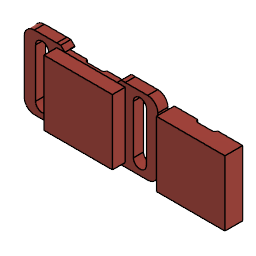
LeverSensor (Autodesk Fusion 360 design; units mm, degrees)
Autodesk Fusion 360 part; units mm, degrees
note: some values were not read from the file. Set by a fixed rule: which sketch regions a step uses.
sketch "Sketch1" plane through (0, 0, 0) normal (0, 0, 1) x (1, 0, 0)
  line L0 (0, 0) -> (12.8, 0)
  line L1 (12.8, 0) -> (12.8, 5.8)
  line L2 (12.8, 5.8) -> (0, 5.8)
  line L3 (0, 5.8) -> (0, 0)
  dimension "d1" = 12.8
  dimension "d2" = 5.8
  constraint horizontal L0
  constraint vertical L1
  constraint horizontal L2
  constraint vertical L3
  constraint coincident L0.start L3.end
  measures "d1" distance of L0.start L0.end
  measures "d2" distance of L0.start L2.end
extrude "Extrude1" add sketch "Sketch1" along normal blind 6 makes body 1
sketch "Sketch2" plane through (0, 0, 0) normal (0, -1, 0) x (1, 0, 0)
  line L0 (0, 0) -> (12.8, 0)
  line L1 (12.8, 0) -> (12.8, 6)
  line L2 (12.8, 6) -> (0, 6)
  line L3 (0, 6) -> (0, 0)
  line L4 (0, 4.8) -> (3.2, 4.8) construction
  circle A0 centre (3.2, 4.8) radius 1.2
  line L5 (6.4, 6) -> (6.4, 0) construction
  circle A1 centre (9.6, 4.8) radius 1.2
  line L6 (1.6, 4.8) -> (4, 4.8)
  line L7 (4, 4.8) -> (4, 6.5)
  line L8 (4, 6.5) -> (1.6, 6.5)
  line L9 (1.6, 6.5) -> (1.6, 4.8)
  line L10 (11.2, 6.5) -> (11.2, 4.8)
  line L11 (11.2, 4.8) -> (8.8, 4.8)
  line L12 (8.8, 4.8) -> (8.8, 6.5)
  line L13 (8.8, 6.5) -> (11.2, 6.5)
  dimension "d5" = 3.2
  dimension "d6" = 2.4
  dimension "d7" = 2.4
  dimension "d8" = 1.7
  constraint coincident L3 L4.start
  constraint perpendicular L3 L4
  constraint coincident L4.end A0.centre
  constraint midpoint L2 L5.start
  constraint midpoint L0 L5.end
  constraint symmetric A0 L5 A1
  constraint horizontal L6
  constraint vertical L7
  constraint horizontal L8
  constraint vertical L9
  constraint midpoint L4 L6.start
  constraint symmetric L5 L6.start L10.end
  constraint symmetric L5 L6.end L11.end
  constraint symmetric L5 L7.end L12.end
  constraint symmetric L5 L8.end L10.start
  measures "d5" distance of L4.start L4.end
  measures "d6" diameter of A0
  measures "d7" distance of L6.start L6.end
  measures "d8" distance of L6.start L8.end
extrude "Extrude2" cut sketch "Sketch2" against normal blind 12 contours A0 L6 L7 | A1 L11 L12 | A0 L6 L7 | A1 L11 L12 bodies 1
extrude "Extrude3" add sketch "Sketch2" against normal blind 5.8 contours L2 L7 L8 L9 | L2 L10 L12 L13 bodies 1
chamfer "Chamfer1" distance 0.5 angle 45 4 edges at (11.2, 2.9, 6.5) (4, 2.9, 6.5) (8.8, 2.9, 6.5) (1.6, 2.9, 6.5) on bodies 1
sketch "Sketch3" plane through (0, 0, 6) normal (0, 0, 1) x (-1, 0, 0)
  line L0 (-8.8, 0) -> (-8.8, -5.8)
  line L1 (-8.8, -5.8) -> (-4, -5.8)
  line L2 (-4, -5.8) -> (-4, 0)
  line L3 (-4, 0) -> (-8.8, 0)
  line L4 (-6.15, -2.65) -> (-6.65, -2.65)
  line L5 (-6.65, -2.65) -> (-6.65, -3.15)
  line L6 (-6.65, -3.15) -> (-6.15, -3.15)
  line L7 (-6.15, -3.15) -> (-6.15, -2.65)
  line L8 (-6.15, -2.65) -> (-6.65, -3.15) construction
  line L9 (-6.65, -2.65) -> (-6.15, -3.15) construction
  line L10 (-11.7603, -2.65) -> (-12.2603, -2.65)
  line L11 (-12.2603, -2.65) -> (-12.2603, -3.15)
  line L12 (-12.2603, -3.15) -> (-11.7603, -3.15)
  line L13 (-11.7603, -3.15) -> (-11.7603, -2.65)
  line L14 (-11.7603, -2.65) -> (-12.2603, -3.15) construction
  line L15 (-12.2603, -2.65) -> (-11.7603, -3.15) construction
  line L16 (-0.6062, -2.65) -> (-1.1062, -2.65)
  line L17 (-1.1062, -2.65) -> (-1.1062, -3.15)
  line L18 (-1.1062, -3.15) -> (-0.6062, -3.15)
  line L19 (-0.6062, -3.15) -> (-0.6062, -2.65)
  line L20 (-0.6062, -2.65) -> (-1.1062, -3.15) construction
  line L21 (-1.1062, -2.65) -> (-0.6062, -3.15) construction
  point P0 (-6.4, -2.9)
  point P1 (-12.0103, -2.9)
  point P2 (-0.8562, -2.9)
  dimension "d14" = 0.5
  dimension "d15" = 0.5
  dimension "d16" = 0.5
  dimension "d17" = 0.5
  dimension "d18" = 0.5
  dimension "d19" = 0.5
  constraint horizontal L4
  constraint perpendicular L4 L5
  constraint parallel L4 L6
  constraint parallel L5 L7
  constraint coincident L8 P0
  constraint coincident L9 P0
  constraint horizontal L10
  constraint perpendicular L10 L11
  constraint parallel L10 L12
  constraint parallel L11 L13
  constraint coincident L14 P1
  constraint coincident L15 P1
  constraint horizontal L16
  constraint perpendicular L16 L17
  constraint parallel L16 L18
  constraint parallel L17 L19
  constraint coincident L20 P2
  constraint coincident L21 P2
  measures "d14" distance of L5.end L6.end
  measures "d15" distance of L4.end L5.end
  measures "d16" distance of L11.end L12.end
  measures "d17" distance of L10.end L11.end
  measures "d18" distance of L17.end L18.end
  measures "d19" distance of L16.end L17.end
extrude "Extrude4" add sketch "Sketch3" along normal blind 5 contours L4 L5 L6 L7 | L10 L11 L12 L13 | L16 L17 L18 L19 bodies 1
sketch "Sketch4" plane through (0, 0, 0) normal (0, -1, 0) x (1, 0, 0)
  circle A0 centre (9.6, 4.8) radius 1.2
  circle A1 centre (3.2, 4.8) radius 1.2
  line L0 (2.1, 6.5) -> (1.6, 6)
  line L1 (1.6, 6) -> (0, 6)
  line L2 (0, 6) -> (0, 0)
  line L3 (0, 0) -> (12.8, 0)
  line L4 (12.8, 0) -> (12.8, 6)
  line L5 (12.8, 6) -> (11.2, 6)
  line L6 (11.2, 6) -> (10.7, 6.5)
  line L7 (10.7, 6.5) -> (9.3, 6.5)
  line L8 (9.3, 6.5) -> (8.8, 6)
  line L9 (8.8, 6) -> (4, 6)
  line L10 (4, 6) -> (3.5, 6.5)
  line L11 (3.5, 6.5) -> (2.1, 6.5)
  circle A2 centre (3.2, 4.8) radius 1
  circle A3 centre (9.6, 4.8) radius 1
  line L12 (0, 0.5) -> (12.8, 0.5)
  line L13 (12.8, 0.5) -> (12.8, 16.5)
  line L14 (12.8, 16.5) -> (0, 16.5)
  line L15 (0, 16.5) -> (0, 0.5)
  line L16 (0, 16.5) -> (-2, 16.5)
  line L17 (-2, 16.5) -> (-2, 0.5)
  line L18 (-2, 0.5) -> (0, 0.5)
  line L19 (0, 0.5) -> (0, 16.5)
  line L20 (12.8, 0.5) -> (14.8, 0.5)
  line L21 (14.8, 0.5) -> (14.8, 16.5)
  line L22 (14.8, 16.5) -> (12.8, 16.5)
  line L23 (12.8, 16.5) -> (12.8, 0.5)
  dimension "d22" = 2
  dimension "d23" = 2
  dimension "d24" = 16
  dimension "d25" = 2
  dimension "d26" = 2
  dimension "d53" = 6.4
  constraint concentric A1 A2
  constraint concentric A0 A3
  constraint horizontal L12
  constraint vertical L13
  constraint horizontal L14
  constraint vertical L15
  constraint coincident L2 L12.start
  constraint horizontal L16
  constraint vertical L17
  constraint horizontal L18
  constraint vertical L19
  constraint horizontal L20
  constraint vertical L21
  constraint horizontal L22
  constraint vertical L23
  measures "d22" diameter of A2
  measures "d23" diameter of A3
  measures "d24" distance of L12.start L14.end
  measures "d25" distance of L14.end L16.end
  measures "d26" distance of L12.end L20.end
  measures "d53" distance of A1.centre A0.centre
extrude "Extrude5" add sketch "Sketch4" along normal blind 1.5 separate body contours A0 | A1 | L0 L1 L2 L4 L5 L6 L7 L8 L9 L10 L11 L12 L13 L15 L19 L23 | L0 L1 L5 L6 L7 L8 L9 L10 L11 L13 L14 L15 L19 L23 | L2 L15 L16 L17 L18 L19 | L4 L13 L20 L21 L22 L23 | A2 | A3 makes body 2
extrude "Extrude6" add sketch "Sketch4" against normal blind 1.5 contours A2 | A3 bodies 2
sketch "Sketch5" plane through (0, 0, 0) normal (0, 1, 0) x (-1, 0, 0)
  circle A0 centre (-9.6, 4.8) radius 1
  circle A1 centre (-3.2, 4.8) radius 1
  line L0 (2, 16.5) -> (-14.8, 16.5)
  line L1 (-14.8, 16.5) -> (-14.8, 0.5)
  line L2 (-14.8, 0.5) -> (2, 0.5)
  line L3 (2, 0.5) -> (2, 16.5)
  line L4 (-14.8, 0.5) -> (-13.5, 0.5)
  line L5 (-13.5, 0.5) -> (-13.5, 15)
  line L6 (-13.5, 16.5) -> (-14.8, 16.5)
  line L7 (-14.8, 16.5) -> (-14.8, 0.5)
  line L8 (2, 0.5) -> (0.7, 0.5)
  line L9 (0.7, 0.5) -> (0.7, 15)
  line L10 (0.2, 16.5) -> (2, 16.5)
  line L11 (2, 16.5) -> (2, 0.5)
  line L12 (-13.5, 16.5) -> (0.2, 16.5)
  line L13 (0.7, 15) -> (-13.5, 15)
  dimension "d31" = 1.3
  dimension "d32" = 1.3
  dimension "d33" = 1.5
  constraint horizontal L4
  constraint vertical L5
  constraint horizontal L6
  constraint vertical L7
  constraint coincident L0 L6.start
  constraint coincident L1.end L2.start
  constraint horizontal L8
  constraint vertical L9
  constraint horizontal L10
  constraint vertical L11
  constraint coincident L0 L10.start
  constraint coincident L2.end L3.start
  constraint horizontal L12
  constraint horizontal L13
  measures "d31" distance of L1.end L4.end
  measures "d32" distance of L2.end L8.end
  measures "d33" distance of L6.start L5.end
extrude "Extrude7" add sketch "Sketch5" along normal blind 2.9 contours L0 L1 L2 L3 L4 L5 L6 L7 L8 L9 L10 L11 L12 L13 bodies 2
mirror "Mirror1" about plane through (0, 2.9, 0) normal (0, 1, 0) of bodies 2 makes body 3
sketch "Sketch6" plane through (0, 2.9, 0) normal (0, 1, 0) x (-1, 0, 0)
  line L0 (2, 16.5) -> (-14.8, 16.5)
  line L1 (-14.8, 16.5) -> (-14.8, 0.5)
  line L2 (-14.8, 0.5) -> (-13.5, 0.5)
  line L3 (-13.5, 0.5) -> (-13.5, 15)
  line L4 (-13.5, 15) -> (0.7, 15)
  line L5 (0.7, 15) -> (0.7, 0.5)
  line L6 (0.7, 0.5) -> (2, 0.5)
  line L7 (2, 0.5) -> (2, 16.5)
  line L8 (-14.8, 16.5) -> (2, 16.5)
  line L9 (2, 16.5) -> (2, 17.5393)
  line L10 (2, 17.5393) -> (-14.8, 17.5393)
  line L11 (-14.8, 17.5393) -> (-14.8, 16.5)
  line L12 (-13.5, 0.5) -> (-14.8, 0.5)
  line L13 (-14.8, 0.5) -> (-14.8, -0.5)
  line L14 (-14.8, -0.5) -> (-13.5, -0.5)
  line L15 (-13.5, -0.5) -> (-13.5, 0.5)
  line L16 (2, 0.5) -> (0.7, 0.5)
  line L17 (0.7, 0.5) -> (0.7, -0.5)
  line L18 (0.7, -0.5) -> (2, -0.5)
  line L19 (2, -0.5) -> (2, 0.5)
  dimension "d38" = 1
  dimension "d39" = 1
  constraint horizontal L8
  constraint vertical L9
  constraint horizontal L10
  constraint vertical L11
  constraint coincident L0.end L1.start
  constraint horizontal L12
  constraint vertical L13
  constraint horizontal L14
  constraint vertical L15
  constraint coincident L2.end L3.start
  constraint horizontal L16
  constraint vertical L17
  constraint horizontal L18
  constraint vertical L19
  constraint coincident L6.end L7.start
  measures "d38" distance of L2.end L14.end
  measures "d39" distance of L6.end L18.end
extrude "Extrude8" add sketch "Sketch6" along normal mid plane 2.5 contours L0 L8 L9 L10 L11 | L6 L16 L17 L18 L19 | L2 L12 L13 L14 L15 bodies 2
sketch "Sketch7" plane through (0, 2.9, 0) normal (0, 1, 0) x (-1, 0, 0)
  line L0 (2, 16.5) -> (-14.8, 16.5)
  line L1 (-14.8, 16.5) -> (-14.8, 0.5)
  line L2 (-14.8, 0.5) -> (-13.5, 0.5)
  line L3 (-13.5, 0.5) -> (-13.5, 15)
  line L4 (-13.5, 15) -> (0.7, 15)
  line L5 (0.7, 15) -> (0.7, 0.5)
  line L6 (0.7, 0.5) -> (2, 0.5)
  line L7 (2, 0.5) -> (2, 16.5)
  line L8 (-14.8, 16.5) -> (1.5, 16.5) construction
  line L9 (1.5, 17.5053) -> (-14.8, 17.5053) construction
  line L10 (-14.8, 17.5053) -> (-14.8, 16.5) construction
  line L11 (-14.8, 17.5053) -> (-20.3, 17.5053)
  line L12 (-22.8, 15.0053) -> (-22.8, 1.9976)
  line L13 (-20.3, -0.5024) -> (-14.8, -0.5024)
  line L14 (-14.8, -0.5024) -> (-14.8, 17.5053)
  line L15 (-6.4, 16.5) -> (-18.4, 16.5) construction
  line L16 (-18.4, 16.5) -> (5.6, 16.5) construction
  line L17 (5.6, 16.5) -> (5.6, 0.5) construction
  line L18 (5.6, 0.5) -> (-18.4, 0.5) construction
  line L19 (-18.4, 0.5) -> (-18.4, 16.5) construction
  line L20 (-16.8, 2.5) -> (-16.8, 14.5)
  arc A0 (-16.8, 14.5) -> (-20, 14.5) centre (-18.4, 14.5) ccw
  line L21 (-20, 14.5) -> (-20, 2.5)
  arc A1 (-20, 2.5) -> (-16.8, 2.5) centre (-18.4, 2.5) ccw
  line L22 (-18.4, 2.5) -> (-18.4, 14.5) construction
  line L23 (-6.4, 16.5) -> (-6.4, 0.5) construction
  arc A2 (-20.3, 17.5053) -> (-22.8, 15.0053) centre (-20.3, 15.0053) ccw
  arc A3 (-22.8, 1.9976) -> (-20.3, -0.5024) centre (-20.3, 1.9976) ccw
  line L24 (7.2, 14.5) -> (7.2, 2.5)
  arc A4 (4, 2.5) -> (7.2, 2.5) centre (5.6, 2.5) ccw
  arc A5 (7.2, 14.5) -> (4, 14.5) centre (5.6, 14.5) ccw
  line L25 (4, 2.5) -> (4, 14.5)
  line L26 (10, 15.0053) -> (10, 1.9976)
  arc A6 (7.5, -0.5024) -> (10, 1.9976) centre (7.5, 1.9976) ccw
  line L27 (7.5, -0.5024) -> (2, -0.5024)
  line L28 (2, -0.5024) -> (2, 17.5053)
  arc A7 (10, 15.0053) -> (7.5, 17.5053) centre (7.5, 15.0053) ccw
  line L29 (2, 17.5053) -> (7.5, 17.5053)
  point P0 (-22.8, 17.5053)
  point P1 (-18.4, 8.5)
  dimension "d44" = 8
  dimension "d45" = 12
  dimension "d46" = 24
  dimension "d48" = 24
  dimension "d49" = 3.2
  dimension "d50" = 2.5
  constraint horizontal L8
  constraint horizontal L9
  constraint vertical L10
  constraint coincident L0.end L1.start
  constraint horizontal L11
  constraint vertical L12
  constraint horizontal L13
  constraint vertical L14
  constraint midpoint L0 L15.start
  constraint parallel L8 L15
  constraint perpendicular L7 L16
  constraint perpendicular L16 L17
  constraint perpendicular L14 L18
  constraint tangent L20 A0
  constraint tangent A0 L21
  constraint parallel L20 L21
  constraint tangent L21 A1
  constraint tangent L20 A1
  constraint coincident L19 A0.centre
  constraint perpendicular L4 L22
  constraint midpoint L19 P1
  constraint midpoint L22 P1
  constraint midpoint L18 L23.end
  constraint coincident P0 L11
  constraint coincident P0 L12
  constraint tangent L11 A2
  constraint tangent L12 A2
  constraint tangent L12 A3
  constraint tangent L13 A3
  constraint equal A2 A3
  constraint symmetric L9.end L23 L28.end
  constraint symmetric L13.end L23 L27.end
  constraint symmetric L20.start L23 A4.start
  constraint symmetric L20.end L23 A5.end
  constraint symmetric A0.end L23 L24.start
  constraint symmetric L21.end L23 L24.end
  constraint symmetric A0 L23 A5
  constraint symmetric A1 L23 A4
  constraint symmetric L23 L11.end A7.end
  constraint symmetric L23 L12.start L26.start
  constraint symmetric L23 A2 A7
  constraint symmetric L23 L12.end L26.end
  constraint symmetric L23 L13.start A6.start
  constraint symmetric L23 A3 A6
  measures "d44" distance of L9.end P0
  measures "d45" distance of L15.start L15.end
  measures "d46" distance of L15.end L16.end
  measures "d48" distance of L17.end L18.end
  measures "d49" diameter of A0
  measures "d50" radius of A2
extrude "Extrude9" add sketch "Sketch7" along normal mid plane 2.5 contours L7 L26 A6 L27 L28 A7 L29 | L1 L11 L12 L13 L14 A2 A3 bodies 2
sketch "Sketch8" plane through (0, 0, 17.5393) normal (0, 0, 1) x (-1, 0, 0)
  line L0 (-14.8, -1.65) -> (-14.8, -4.15)
  line L1 (-14.8, -4.15) -> (2, -4.15)
  line L2 (2, -4.15) -> (2, -1.65)
  line L3 (2, -1.65) -> (-14.8, -1.65)
  line L4 (-8.4, -3.55) -> (-4.9, -3.55)
  arc A0 (-4.9, -3.55) -> (-4.9, -2.25) centre (-4.9, -2.9) ccw
  line L5 (-4.9, -2.25) -> (-8.4, -2.25)
  arc A1 (-8.4, -2.25) -> (-8.4, -3.55) centre (-8.4, -2.9) ccw
  line L6 (-8.4, -2.9) -> (-4.9, -2.9) construction
  point P0 (-6.65, -2.9)
  dimension "d54" = 1.3
  constraint tangent L4 A0
  constraint tangent A0 L5
  constraint parallel L4 L5
  constraint tangent L5 A1
  constraint tangent L4 A1
  constraint perpendicular L0 L6
  constraint midpoint L6 P0
  measures "d54" diameter of A0
extrude "Extrude10" cut sketch "Sketch8" against normal blind 7 contours L4 A0 L5 A1 bodies 2 3
sketch "Sketch9" plane through (0, 0, 17.5393) normal (0, 0, 1) x (-1, 0, 0)
  line L0 (-4.9, -3.55) -> (-8.4, -3.55)
  arc A0 (-8.4, -2.25) -> (-8.4, -3.55) centre (-8.4, -2.9) ccw
  line L1 (-8.4, -2.25) -> (-4.9, -2.25)
  arc A1 (-4.9, -3.55) -> (-4.9, -2.25) centre (-4.9, -2.9) ccw
  line L2 (-14.8, -1.65) -> (-14.8, -4.15)
  line L3 (-14.8, -4.15) -> (2, -4.15)
  line L4 (2, -4.15) -> (2, -1.65)
  line L5 (2, -1.65) -> (-14.8, -1.65)
  line L6 (-14.8, -1.65) -> (-12.8, -1.65) construction
  line L7 (-12.8, -1.65) -> (-12.8, -4.15) construction
  line L8 (-12.8, -4.15) -> (-14.8, -4.15) construction
  line L9 (-14.8, -4.15) -> (-14.8, -1.65) construction
  line L10 (2, -1.65) -> (0, -1.65) construction
  line L11 (0, -1.65) -> (0, -4.15) construction
  line L12 (0, -4.15) -> (2, -4.15) construction
  line L13 (2, -4.15) -> (2, -1.65) construction
  line L14 (-12.8, -1.65) -> (0, -1.65)
  line L15 (0, -1.65) -> (0, -4.15)
  line L16 (0, -4.15) -> (-12.8, -4.15)
  line L17 (-12.8, -4.15) -> (-12.8, -1.65)
  dimension "d60" = 2
  dimension "d61" = 2
  constraint horizontal L6
  constraint vertical L7
  constraint horizontal L8
  constraint vertical L9
  constraint coincident L2.start L5.end
  constraint horizontal L10
  constraint vertical L11
  constraint horizontal L12
  constraint vertical L13
  constraint coincident L4.end L5.start
  constraint horizontal L14
  constraint vertical L15
  constraint horizontal L16
  constraint vertical L17
  measures "d60" distance of L2.start L6.end
  measures "d61" distance of L4.end L10.end
extrude "Extrude12" cut sketch "Sketch9" against normal blind 1.039 contours L3 L5 L14 L15 L16 L17 bodies 2
extrude "Extrude13" cut 2 faces at (13.4667, 2.4833, 17.5393) (-1.3333, 2.4833, 17.5393) along direction (0, 0, -1) blind 0.034 on bodies 2 bodies 2
chamfer "Chamfer3" distance 1 angle 45 2 edges at (12.8, 2.9, 17.5053) (0, 2.9, 17.5053) on bodies 2
move_body "Move1" bodies 3 to x (-1, 0, 0) y (0, -1, 0) z (0, 0, 1) at (39.6, 6.6, 0)
extrude "Extrude14" cut 1 faces at (0.0855, 3.3475, 16.5) along direction (0, 0, 1) blind 0.05 on bodies 2 bodies 2
extrude "Extrude15" add 2 faces at (13.4964, 3.7333, 16.55) (-0.6964, 3.3167, 16.55) along direction (0, 0, -1) blind 0.15 on bodies 2 bodies 2
hidden bodies 1
equation "d5 = 2.4 mm + 0.8 mm"
equation "d8 = 1.2 mm + 0.5 mm"
equation "d51 = -2.5 * 0.5 mm"
